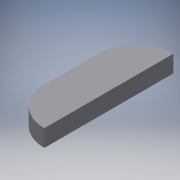
# Autodesk Inventor part: waterbottle_holder_side
Saved by Autodesk Inventor 2017.2 (Build 212233000, 233)
## iProperties
Created: 2017-09-01
Part Number: waterbottle_holder_side
Material: Generic
Document SubType Name: Modeling
Designer: Nic
Density: 1 g/cm^3
Appearance: Default
Author: Nic
Autodesk Inventor part; units mm, degrees
ref_plane "YZ Plane" through (0, 0, 0) normal (1, 0, 0) x (0, 1, 0)
ref_plane "XZ Plane" through (0, 0, 0) normal (0, 1, 0) x (-1, 0, 0)
ref_plane "XY Plane" through (0, 0, 0) normal (0, 0, 1) x (1, 0, 0)
sketch "Sketch1" plane through (0, 0, 0) normal (0, 0, 1) x (1, 0, 0)
  line L0 (0, 0) -> (-7, 0) construction
  line L1 (-7, 0) -> (-7, 5)
  arc A0 (0, 12) -> (-7, 5) centre (0, 5) ccw
  line L2 (0, 12) -> (0, 0)
  line L3 (-7, 0) -> (-7, -5)
  arc A1 (-7, -5) -> (0, -12) centre (0, -5) ccw
  line L4 (0, -12) -> (0, 0)
  dimension "d0" = 7
  dimension "d2" = 7
  dimension "d5" = 5
  constraints: 10 end point, 4 point on circle, 3 symmetric about line, 2 centre point, 1 horizontal, 1 parallel, 1 tangent, 1 vertical, 1 other
  measures "d0" radius of A0
  measures "d2" distance of L0.start L0.end
  measures "d5" distance of L0.end L1.end
extrude "Extrusion1" add sketch "Sketch1" along normal blind 3.175
body "Solid1"
